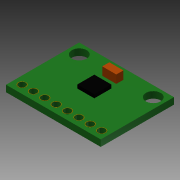
# Autodesk Inventor part: GY-521 Gyro
Saved by Autodesk Inventor 2014 (Build 180170000, 170)
## iProperties
Created: 2014-03-02
Part Number: GY-521 Gyro
Material: Generic
Document SubType Name: Modeling
Designer: Spooner
Density: 1 g/cm^3
Appearance: Smooth - Dark Forest Green
Author: Spooner
Autodesk Inventor part; units mm, degrees
ref_plane "YZ Plane" through (0, 0, 0) normal (1, 0, 0) x (0, 1, 0)
ref_plane "XZ Plane" through (0, 0, 0) normal (0, 1, 0) x (-1, 0, 0)
ref_plane "XY Plane" through (0, 0, 0) normal (0, 0, 1) x (1, 0, 0)
sketch "Sketch1" plane through (0, 0, 0) normal (0, 1, 0) x (-1, 0, 0)
  line L0 (0, 0) -> (21.1582, 0)
  line L1 (21.1582, 0) -> (21.1582, 16.3576)
  line L2 (21.1582, 16.3576) -> (0, 16.3576)
  line L3 (0, 16.3576) -> (0, 0)
  dimension "d0" = 21.1582
  dimension "d1" = 16.3576
  constraints: 8 end point, 2 parallel, 1 horizontal, 1 perpendicular
  measures "d0" distance of L0.start L0.end
  measures "d1" distance of L2.end L0.start
extrude "Extrusion1" add sketch "Sketch1" along normal blind 1.4478
sketch "Sketch2" plane through (0, 1.4478, 0) normal (0, 1, 0) x (1, 0, 0)
  line L0 (0, 0) -> (-21.1582, 0) projected
  line L1 (-21.1582, 0) -> (-21.1582, -16.3576) projected
  line L2 (0, -16.3576) -> (0, 0) projected
  circle A0 centre (-18.8468, -2.3114) radius 1.651
  circle A1 centre (-2.3114, -2.3114) radius 1.651
  dimension "d4" = 0.6604
  dimension "d5" = 0.6604
  dimension "d6" = 0.6604
  dimension "d7" = 3.302
  constraints: 2 centre point, 1 equal radius, 1 horizontal alignment
  measures "d4" distance edge to line of A0 L0
  measures "d5" distance edge to line of A0 L1
  measures "d6" distance edge to line of A1 L2
  measures "d7" diameter of A1
extrude "Extrusion2" cut sketch "Sketch2" against normal through all
sketch "Sketch3" plane through (0, 1.4478, 0) normal (0, 1, 0) x (1, 0, 0)
  line L0 (0, 0) -> (-21.1582, 0) projected
  line L1 (-12.1539, -2.286) -> (-9.0043, -2.286)
  line L2 (-9.0043, -2.286) -> (-9.0043, -3.8735)
  line L3 (-9.0043, -3.8735) -> (-12.1539, -3.8735)
  line L4 (-12.1539, -3.8735) -> (-12.1539, -2.286)
  point P0 (-10.5791, -2.286)
  point P1 (-10.5791, 0)
  dimension "d10" = 3.1496
  dimension "d11" = 1.5875
  dimension "d12" = 2.286
  constraints: 8 end point, 2 midpoint, 2 parallel, 2 vertical alignment, 1 horizontal, 1 perpendicular
  measures "d10" distance of L1.start L1.end
  measures "d11" distance of L3.end L1.start
  measures "d12" distance between parallel lines of L1 L0
extrude "Extrusion3" add sketch "Sketch3" along normal blind 1.8161
sketch "Sketch4" plane through (0, 1.4478, 0) normal (0, 1, 0) x (1, 0, 0)
  line L0 (-9.0043, -3.8735) -> (-12.1539, -3.8735) projected
  line L1 (0, 0) -> (-21.1582, 0) projected
  line L2 (-8.6741, -5.3086) -> (-12.4841, -5.3086)
  line L3 (-12.4841, -5.3086) -> (-12.4841, -9.1186)
  line L4 (-12.4841, -9.1186) -> (-8.6741, -9.1186)
  line L5 (-8.6741, -9.1186) -> (-8.6741, -5.3086)
  line L6 (-8.6741, -5.3086) -> (-12.4841, -9.1186) construction
  line L7 (-12.4841, -5.3086) -> (-8.6741, -9.1186) construction
  point P0 (-10.5791, -7.2136)
  point P1 (-10.5791, 0)
  point P2 (-10.5791, -7.2136)
  dimension "d15" = 3.81
  dimension "d16" = 3.81
  dimension "d17" = 1.4351
  constraints: 12 end point, 4 midpoint, 2 parallel, 1 horizontal, 1 perpendicular, 1 vertical alignment
  measures "d15" distance of L2.end L3.end
  measures "d16" distance of L2.start L2.end
  measures "d17" distance between parallel lines of L2 L0
extrude "Extrusion4" add sketch "Sketch4" along normal blind 0.762
sketch "Sketch5" plane through (0, 1.4478, 0) normal (0, 1, 0) x (1, 0, 0)
  line L0 (-21.1582, 0) -> (-21.1582, -16.3576) projected
  line L1 (-21.1582, -16.3576) -> (0, -16.3576) projected
  circle A0 centre (-19.3662, -14.5656) radius 0.776
  dimension "d20" = 1.016
  dimension "d21" = 1.016
  constraints: 1 centre point
  measures "d20" distance edge to line of A0 L1
  measures "d21" distance edge to line of A0 L0
extrude "Extrusion5" cut sketch "Sketch5" against normal through all
sketch "Sketch6" plane through (0, 1.4478, 0) normal (0, 1, 0) x (1, 0, 0)
  circle A0 centre (-19.3662, -14.5656) radius 0.776 projected
  circle A1 centre (-19.3662, -14.5656) radius 0.889
  dimension "d24" = 1.778
  constraints: 1 centre point, 1 coincident
  measures "d24" diameter of A1
extrude "Extrusion6" add sketch "Sketch6" along normal blind 0.0254
pattern_linear "Rectangular Pattern1" count 8 spacing 2.54 along (1, 0, 0) of "Extrusion5", "Extrusion6"
equation "\"d5\" = d4"
equation "\"d6\" = d5"
body "Solid1"
